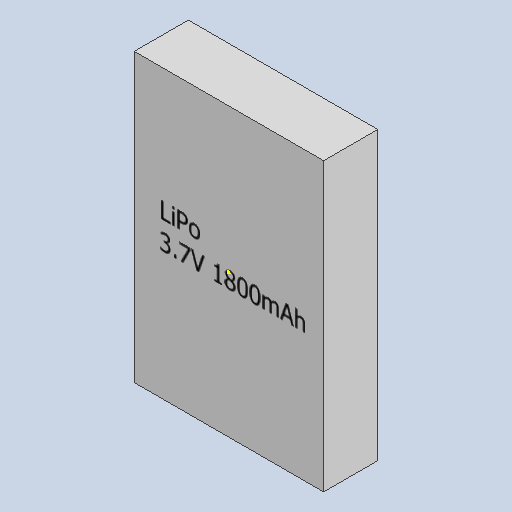
# Autodesk Inventor part: LiPo-1800mAh
Saved by Autodesk Inventor 2025 (Build 290162000, 162)
## iProperties
Created: 2025-05-29
Part Number: LiPo-1800mAh
Material: 一般
Document SubType Name: Modeling
Designer: yamashita1
Density: 1 g/cm^3
Appearance: 既定
Author: yamashita1
Autodesk Inventor part; units mm, degrees
ref_plane "YZ Plane" through (0, 0, 0) normal (1, 0, 0) x (0, 1, 0)
ref_plane "XZ Plane" through (0, 0, 0) normal (0, 1, 0) x (-1, 0, 0)
ref_plane "XY Plane" through (0, 0, 0) normal (0, 0, 1) x (1, 0, 0)
sketch "スケッチ1" plane through (0, 0, 0) normal (0, 0, 1) x (1, 0, 0)
  line L0 (-17.5, 26.5) -> (17.5, 26.5)
  line L1 (17.5, 26.5) -> (17.5, -26.5)
  line L2 (17.5, -26.5) -> (-17.5, -26.5)
  line L3 (-17.5, -26.5) -> (-17.5, 26.5)
  point P0 (0, 0)
  point P1 (-17.5, 0)
  point P2 (0, 26.5)
  dimension "d0" = 35
  dimension "d1" = 53
  constraints: 8 end point, 2 midpoint, 2 parallel, 1 horizontal, 1 horizontal alignment, 1 perpendicular, 1 vertical alignment
  measures "d0" distance of L1.end L2.end
  measures "d1" distance of L0.end L1.end
extrude "押し出し1" add sketch "スケッチ1" along normal blind 10
sketch "スケッチ2" plane through (0, 0, 10) normal (0, 0, 1) x (1, 0, 0)
  line L0 (-12.853, 5.2467) -> (23.2611, 5.2467) construction
  line L1 (23.2611, 5.2467) -> (23.2611, 1.9936) construction
  line L2 (23.2611, 1.9936) -> (-12.853, 1.9936) construction
  line L3 (-12.853, 1.9936) -> (-12.853, 5.2467) construction
  point P0 (0, 0)
  constraints: 2 other
